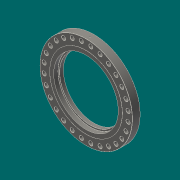
# Autodesk Inventor part: A1-19010-100-01 30in CL300 RFBL flange
Saved by Autodesk Inventor 2017.3 (Build 213257000, 257)
## iProperties
Created: 2019-09-04
Part Number: A1-19010-100-01 30in CL300 RFBL flange
Material: A105N
Document SubType Name: Modeling
Designer: Graeme_Van_Dongen
Density: 7.85 g/cm^3
Appearance: Steel - Cast
Mass: 332602 g
Surface Area: 18798.6 cm^2
Volume: 42369.7 cm^3
Description: Ø30" CLASS 300 RFBL FLANGE, A105N, ASME B16.47 Ser.A - CUSTOM
od: 43.000 in
bore: 28 1/2"
Author: JDS
Autodesk Inventor part; units mm, degrees
ref_plane "YZ Plane" through (0, 0, 0) normal (1, 0, 0) x (0, 1, 0)
ref_plane "XY Plane" through (0, 0, 0) normal (0, 0, 1) x (1, 0, 0)
sketch "Sketch1" plane through (0, 0, 0) normal (0, 0, 1) x (1, 0, 0)
  circle A0 centre (0, 0) radius 546.1
  dimension "d0" = 1092.2
  constraints: 1 centre point, 1 coincident
  measures "d0" diameter of A0
extrude "Extrusion: OD" add sketch "Sketch1" along normal blind 93.4125
sketch "Sketch2" plane through (0, 0, 93.4125) normal (0, 0, 1) x (1, 0, 0)
  circle A0 centre (0, 0) radius 428.625
  dimension "d3" = 857.25
  constraints: 1 centre point, 1 coincident
  measures "d3" diameter of A0
extrude "Extrusion: RF" add sketch "Sketch2" along normal blind 1.5875
sketch "Sketch3" plane through (0, 0, 95) normal (0, 0, 1) x (1, 0, 0)
  circle A0 centre (0, 0) radius 381
  dimension "d6" = 762
  dimension "d32" = 0
  constraints: 1 centre point, 1 coincident
  measures "d6" diameter of A0
  measures "d32" distance of point (0, 0) A0.centre
extrude "Extrusion: ID Large" cut sketch "Sketch3" against normal blind 50.8
sketch "Sketch4" plane through (0, 0, 95) normal (0, 0, 1) x (1, 0, 0)
  circle A0 centre (0, 0) radius 361.95
  circle A1 centre (0, 0) radius 428.625 projected
  dimension "bore" = 723.9
  constraints: 1 centre point, 1 coincident
  measures "bore" diameter of A0
extrude "Extrusion: ID Small" cut sketch "Sketch4" along normal through all both and the other way through all contours A0
sketch "Sketch5" plane through (0, 0, 95) normal (0, 0, 1) x (1, 0, 0)
  line L0 (-495.3407, -55.8115) -> (495.3407, 55.8115)
  line L1 (-495.3407, -55.8115) -> (501.6093, -55.8115) construction
  point P0 (0, 0)
  point P1 (0, 0)
  dimension "d12" = 996.95
  dimension "d13" = 6.429
  constraints: 4 end point, 2 coincident, 1 equal length, 1 horizontal, 1 midpoint
  measures "d12" distance of L0.start L0.end
  measures "d13" angle of L1 L0
hole "Hole: Bolt" at (495.3407, 55.8115, 95) direction (0, 0, -1) diameter 47.625 end through all
chamfer "Chamfer: Bolt hole" distance 1.5875 angle 45 2 edges at (495.3407, 79.624, 93.4125) (495.3407, 79.624, 0)
pattern_circular "Circular Pattern: Bolt hole" count 28 over 360 about axis through (0, 0, -10) along (0, 0, 1) of "Hole: Bolt", "Chamfer: Bolt hole"
chamfer "Chamfer: OD" distance 1.5875 angle 45 2 edges at (-546.1, 0, 93.4125) (-546.1, 0, 0)
chamfer "Chamfer2" distance 0.7937 angle 45 1 edges at (-361.95, 0, 44.2)
fillet "Fillet2" radius 0.7937 1 edges at (-381, 0, 44.2)
ref_plane "Work Plane1" through (0, 546.1, 0) normal (0, 1, 0) x (-1, 0, 0)
sketch "Sketch6" plane through (0, 546.1, 0) normal (0, 1, 0) x (-1, 0, 0)
  point P0 (0, 0)
  point P1 (0, 47.5)
  dimension "d36" = 47.5
  constraints: 1 vertical alignment
  measures "d36" distance of point (0, 0) point (0, 47.5)
hole "Hole2" at (0, 546.1, 47.5) direction (0, -1, 0) diameter 16.3068 depth 63.5 tip angle 118 thread size "3/4-10 UNC" class "2B" standard "ANSI Unified Screw Threads"
pattern_circular "Circular Pattern2" count 2 over 360 about axis through (0, 0, -10) along (0, 0, 1) of "Hole2"
equation "\"d0\" = od"
equation "\"d1\" = thk - rf"
equation "\"d3\" = od_rf"
equation "\"d4\" = rf"
equation "\"d6\" = cbore"
equation "\"bore\" = cbore - 2 * r_diff_cbore"
equation "\"d36\" = 0.5 * d4 + 0.5 * d1"
equation "\"od\" = 1092.2"
equation "\"thk\" = 95"
equation "\"rf\" = 1.5875"
equation "\"od_rf\" = 857.25"
equation "\"cbore\" = 762"
equation "\"r_diff_cbore\" = 19.05"
body "Solid1"
